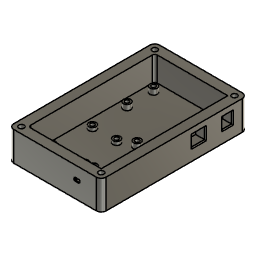
Smart Lock Enclosure Base v9 (Autodesk Fusion 360 design; units mm, degrees)
Autodesk Fusion 360 part; units mm, degrees
sketch "Sketch1" plane through (0, 0, 0) normal (0, 0, 1) x (1, 0, 0)
  line L0 (47.5, 75) -> (-47.5, 75)
  line L1 (-47.5, 75) -> (-47.5, -75)
  line L2 (-47.5, -75) -> (47.5, -75)
  line L3 (47.5, -75) -> (47.5, 75)
  line L4 (47.5, 75) -> (-47.5, -75) construction
  line L5 (-47.5, 75) -> (47.5, -75) construction
  dimension "d1" = 95
  dimension "d2" = 150
  constraint horizontal L0
  constraint perpendicular L0 L1
  constraint parallel L0 L2
  constraint parallel L1 L3
  constraint coincident L4 origin
  constraint coincident L5 origin
  measures "d1" distance of L1.end L2.end
  measures "d2" distance of L0.end L1.end
extrude "Extrude1" add sketch "Sketch1" along normal blind 30 makes body 1
fillet "Fillet1" radius 5 1 edges at (47.5, -75, 15) on bodies 1
fillet "Fillet2" radius 5 1 edges at (47.5, 75, 15) on bodies 1
fillet "Fillet3" radius 5 1 edges at (-47.5, 75, 15) on bodies 1
fillet "Fillet4" radius 5 1 edges at (-47.5, -75, 15) on bodies 1
shell "Shell1" thickness 10 removed faces 1 at (-15.8333, -23.3333, 30) on bodies 1
fillet "Fillet7" radius 2.5 1 edges at (-37.5, -65, 20) on bodies 1
fillet "Fillet8" radius 2.5 1 edges at (-37.5, 65, 20) on bodies 1
hole "Hole1" at (41, -68.5, 0) direction (0, 0, 1) diameter 5.5 depth 30 tip angle 180 countersink diameter 10 countersink angle 90 bodies 1
hole "Hole2" at (-41, -68.5, 0) direction (0, 0, 1) diameter 5.5 depth 30 tip angle 180 countersink diameter 10 countersink angle 90 bodies 1
hole "Hole3" at (-41, 68.5, 0) direction (0, 0, 1) diameter 5.5 depth 30 tip angle 180 countersink diameter 10 countersink angle 90 bodies 1
hole "Hole4" at (41, 68.5, 0) direction (0, 0, 1) diameter 5.5 depth 30 tip angle 180 countersink diameter 10 countersink angle 90 bodies 1
extrude "Extrude2" cut 1 faces at (12.5, 20.8333, 10) along direction (0, 0, -1) blind 5 on bodies 1 bodies 1
box "BoxPrimitive1" cut length 11.5 width 9.5 height -10 placed x (0, 0, 1) y (0, -1, 0) z (1, 0, 0) at (47.5, 59.5, 8.5) bodies 1
move_face "MoveFace1" by (0, 0, 3.5) 1 faces at (40.8333, 56.3333, 8.5) on bodies 1
move_face "MoveFace2" by (0, 0, 3.5) 1 faces at (40.8333, 56.3333, 20) on bodies 1
box "BoxPrimitive2" cut length 11.5 width 13.5 height -10 placed x (0, 0, 1) y (0, -1, 0) z (1, 0, 0) at (47.5, 28.5, 8.5) bodies 1
move_face "MoveFace3" by (0, 0, 3.5) 1 faces at (40.8333, 24, 8.5) on bodies 1
move_face "MoveFace4" by (0, 0, 3.5) 1 faces at (40.8333, 24, 20) on bodies 1
move_face "MoveFace5" by (0, 3.5, 0) 1 faces at (40.8333, 28.5, 19.6667) on bodies 1
move_face "MoveFace6" by (0, 3.5, 0) 1 faces at (40.8333, 15, 19.6667) on bodies 1
cylinder "CylinderPrimitive1" add diameter 7.5 height 5.5 placed x (1, 0, 0) y (0, 1, 0) z (0, 0, 1) at (20, 60, 5) separate body makes body 2
move_body "Move2" bodies 2 to x (1, 0, 0) y (0, 1, 0) z (0, 0, 1) at (1.1, -0.25, 0)
move_body "Move3" bodies 2 to x (1, 0, 0) y (0, 1, 0) z (0, 0, 1) at (2.5, 1, 0)
hole "Hole6" at (23.6, 60.75, 10.5) direction (0, 0, -1) diameter 4.2 depth 6 tip angle 180 bodies 1 2
cylinder "CylinderPrimitive3" add diameter 7.5 height 5.5 placed x (1, 0, 0) y (0, 1, 0) z (0, 0, 1) at (-3, 52, 5) separate body makes body 3
move_body "Move9" bodies 3 to x (1, 0, 0) y (0, 1, 0) z (0, 0, 1) at (0, 3, 0)
move_body "Move10" bodies 3 to x (1, 0, 0) y (0, 1, 0) z (0, 0, 1) at (-25.7, 0, 0)
hole "Hole7" at (-28.7, 55, 10.5) direction (0, 0, -1) diameter 4.2 depth 6 tip angle 180 bodies 1 3
cylinder "CylinderPrimitive4" add diameter 7.5 height 5.5 placed x (1, 0, 0) y (0, 1, 0) z (0, 0, 1) at (-30.517, 18.5394, 5) separate body makes body 4
move_body "Move11" bodies 4 to x (1, 0, 0) y (0, 1, 0) z (0, 0, 1) at (2, 8.961, 0)
hole "Hole8" at (-28.517, 27.5004, 10.5) direction (0, 0, -1) diameter 4.2 depth 6 tip angle 180 bodies 1 4
move_face "MoveFace7" by (0, -0.25, 0) 1 faces at (40.8333, 50, 19.6667) on bodies 1
move_face "MoveFace8" by (0, 0.25, 0) 1 faces at (40.8333, 59.5, 19.6667) on bodies 1
cylinder "CylinderPrimitive5" add diameter 7.5 height 3.5 placed x (1, 0, 0) y (0, 1, 0) z (0, 0, 1) at (-24.3026, -54.6072, 5) separate body makes body 5
move_body "Move13" bodies 5 to x (1, 0, 0) y (0, 1, 0) z (0, 0, 1) at (-8.147, 8.357, 0)
cylinder "CylinderPrimitive6" add diameter 7.5 height 3.5 placed x (1, 0, 0) y (0, 1, 0) z (0, 0, 1) at (-7.6761, -50.1234, 5) separate body makes body 6
move_body "Move14" bodies 6 to x (1, 0, 0) y (0, 1, 0) z (0, 0, 1) at (9.426, 3.873, 0)
cylinder "CylinderPrimitive7" add diameter 7.5 height 3.5 placed x (1, 0, 0) y (0, 1, 0) z (0, 0, 1) at (-30, -20, 5) separate body makes body 7
move_body "Move15" bodies 7 to x (1, 0, 0) y (0, 1, 0) z (0, 0, 1) at (2.25, 11.25, 0)
cylinder "CylinderPrimitive8" add diameter 7.5 height 3.5 placed x (1, 0, 0) y (0, 1, 0) z (0, 0, 1) at (0, -10, 5) separate body makes body 8
move_body "Move16" bodies 8 to x (1, 0, 0) y (0, 1, 0) z (0, 0, 1) at (-2.95, 1.25, 0)
cylinder "CylinderPrimitive9" add diameter 7.5 height 5.5 placed x (1, 0, 0) y (0, 1, 0) z (0, 0, 1) at (30.6169, -3.0137, 5) separate body makes body 9
move_body "Move17" bodies 9 to x (1, 0, 0) y (0, 1, 0) z (0, 0, 1) at (1.433, 5.963, 0)
cylinder "CylinderPrimitive10" add diameter 7.5 height 5.5 placed x (1, 0, 0) y (0, 1, 0) z (0, 0, 1) at (12.5548, -16.5521, 5) separate body makes body 10
move_body "Move18" bodies 10 to x (1, 0, 0) y (0, 1, 0) z (0, 0, 1) at (-1.105, 19.501, 0)
cylinder "CylinderPrimitive11" add diameter 7.5 height 5.5 placed x (1, 0, 0) y (0, 1, 0) z (0, 0, 1) at (32.4744, -42.8025, 5) separate body makes body 11
move_body "Move19" bodies 11 to x (1, 0, 0) y (0, 1, 0) z (0, 0, 1) at (-0.424, 0.752, 0)
cylinder "CylinderPrimitive12" add diameter 7.5 height 5.5 placed x (1, 0, 0) y (0, 1, 0) z (0, 0, 1) at (16.8622, -43.3795, 5) separate body makes body 12
move_body "Move20" bodies 12 to x (1, 0, 0) y (0, 1, 0) z (0, 0, 1) at (-5.412, 1.329, 0)
fillet "Fillet10" radius 1 8 edges at (47.5, 18.5, 17.75) (47.5, 25.25, 23.5) (47.5, 32, 17.75) (47.5, 25.25, 12) (47.5, 54.75, 23.5) (47.5, 49.75, 17.75) (47.5, 54.75, 12) (47.5, 59.75, 17.75) on bodies 1
box "BoxPrimitive18" cut length 2.5 width 5 height -10 placed x (0, 0, 1) y (1, 0, 0) z (0, 1, 0) at (20, -65, 16) bodies 1
fillet "Fillet11" radius 0.5 4 faces at (20, -71.6667, 17.6667) (21.6667, -71.6667, 18.5) (21.6667, -71.6667, 16) (25, -71.6667, 17.6667) on bodies 1
move_body "Move26" bodies 11 12 10 9 to x (1, 0, 0) y (0, 1, 0) z (0, 0, 1) at (0, -5, 0)
hole "Hole17" at (32.0504, -47.0505, 10.5) direction (0, 0, -1) diameter 4.2 depth 6 tip angle 180 bodies 1 11
hole "Hole18" at (11.4502, -47.0505, 10.5) direction (0, 0, -1) diameter 4.2 depth 6 tip angle 180 bodies 1 12
hole "Hole19" at (32.0499, -2.0507, 10.5) direction (0, 0, -1) diameter 4.2 depth 6 tip angle 180 bodies 1 9
hole "Hole20" at (11.4498, -2.0511, 10.5) direction (0, 0, -1) diameter 4.2 depth 6 tip angle 180 bodies 1 10
hole "Hole21" at (1.7499, -46.2504, 8.5) direction (0, 0, -1) diameter 4.2 depth 6 tip angle 180 bodies 1 6
hole "Hole22" at (-2.95, -8.75, 8.5) direction (0, 0, -1) diameter 4.2 depth 6 tip angle 180 bodies 1 8
hole "Hole23" at (-32.4496, -46.2502, 8.5) direction (0, 0, -1) diameter 4.2 depth 6 tip angle 180 bodies 1 5
hole "Hole24" at (-27.75, -8.75, 8.5) direction (0, 0, -1) diameter 4.2 depth 6 tip angle 180 bodies 1 7
